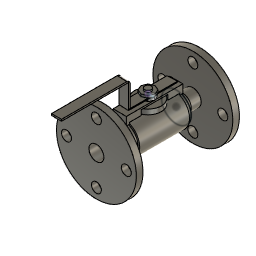
drawing 3 (pipe with handle) v5 (Autodesk Fusion 360 design; units mm, degrees)
Autodesk Fusion 360 part; units mm, degrees
sketch "Sketch1" plane through (0, 0, 0) normal (0, 0, 1) x (1, 0, 0)
  line L0 (0, -75) -> (0, 75)
  constraint vertical L0
pipe "Pipe1" add diameter 100 wall 5 path "Sketch1" along L0 makes body 1
sketch "Sketch2" plane through (0, 75, 0) normal (0, 1, 0) x (-1, 0, 0)
  circle A0 centre (0, 0) radius 45
  circle A1 centre (0, 0) radius 50
  circle A2 centre (0, 0) radius 45
  constraint coincident A0.centre A1.centre
extrude "Extrude1" add sketch "Sketch2" along normal blind 10 separate body contours A0 A2 makes body 2
sketch "Sketch3" plane through (0, 85, 0) normal (0, 1, 0) x (-1, 0, 0)
  circle A0 centre (0, 0) radius 45
  circle A1 centre (0, 0) radius 44
  dimension "d7" = 88
  constraint concentric A0 A1
  measures "d7" diameter of A1
hole "Hole1" at (0, 85, 0) direction (0, -1, 0) diameter 88 depth 40 tip angle 118 bodies 2
mirror "Mirror1" about plane through (0, 0, 0) normal (0, 1, 0) of "Extrude1" makes body 3
ref_plane "WorkPlane1" through (0, -85, 0) normal (0, 1, 0) x (0, 0, 1)
sketch "Sketch4" plane through (0, -85, 0) normal (0, -1, 0) x (1, 0, 0)
  circle A0 centre (0, 0) radius 45
  circle A1 centre (0, 0) radius 25
  dimension "d14" = 50
  constraint coincident A0.centre A1.centre
  measures "d14" diameter of A1
extrude "Extrude2" add sketch "Sketch4" along normal blind 50 contours A1 bodies 3
fillet "Fillet1" radius 20 1 edges at (-23.3082, -85, 9.0404) on bodies 3
ref_plane "WorkPlane2" through (0, -135, 0) normal (0, 1, 0) x (0, 0, 1)
hole "Hole2" at (0, -135, 0) direction (0, 1, 0) diameter 45 depth 60 tip angle 180 bodies 3
sketch "Sketch5" plane through (0, -135, 0) normal (0, 1, 0) x (1, 0, 0)
  circle A0 centre (0, 0) radius 120
  constraint coincident A0.centre origin
extrude "Extrude3" add sketch "Sketch5" against normal blind 20 bodies 3
hole "Hole3" at (0, -155, 0) direction (0, 1, 0) diameter 45 depth 20 tip angle 180 bodies 3
mirror "Mirror2" about plane through (0, 0, 0) normal (0, 1, 0) of bodies 3 makes body 4
sketch "Sketch6" plane through (0, 155, 0) normal (0, 1, 0) x (-1, 0, 0)
  circle A0 centre (0, 0) radius 22.5
  circle A1 centre (0, 0) radius 120
  circle A2 centre (0, 0) radius 90
  line L0 (0, 0) -> (90, 0)
  line L1 (0, 0) -> (0, 90)
  circle A3 centre (0, 90) radius 15
  circle A4 centre (90, 0) radius 15
  circle A5 centre (-90, 0) radius 15
  circle A6 centre (0, -90) radius 15
  dimension "d30" = 180
  dimension "d32" = 30
  dimension "d33" = 30
  dimension "d34" = 30
  dimension "d35" = 30
  constraint concentric A0 A2
  constraint coincident A0.centre A1.centre
  constraint coincident A2 L0.end
  constraint horizontal L0
  constraint coincident A2 L1.end
  constraint perpendicular L0 L1
  constraint coincident L1.end A3.centre
  constraint coincident L0.end A4.centre
  constraint coincident A2 A5.centre
  constraint coincident A2 A6.centre
  measures "d30" diameter of A2
  measures "d32" diameter of A3
  measures "d33" diameter of A4
  measures "d34" diameter of A5
  measures "d35" diameter of A6
extrude "Extrude4" cut sketch "Sketch6" against normal blind 20 contours A2 L0 A4 | A2 L0 A4 | A2 L1 A3 | A2 L1 A3 | A2 A4 | A2 A3 | A2 A6 | A2 A6 | A2 A5 | A2 A5 bodies 4
mirror "Mirror3" about plane through (0, 0, 0) normal (0, 1, 0) of "Extrude4"
mirror "Mirror4" about plane through (0, 0, 0) normal (0, 1, 0) of "Extrude4"
mirror "Mirror5" about plane through (0, 0, 0) normal (0, 1, 0) of "Extrude4"
sketch "Sketch7" plane through (0, -155, 0) normal (0, -1, 0) x (1, 0, 0)
  circle A0 centre (0, 0) radius 22.5
  circle A1 centre (0, 0) radius 120
  circle A2 centre (0, 0) radius 90
  circle A3 centre (0, 90) radius 15
  circle A4 centre (90, 0) radius 15
  circle A5 centre (0, -90) radius 15
  circle A6 centre (-90, 0) radius 15
  dimension "d44" = 180
  dimension "d45" = 30
  dimension "d46" = 30
  dimension "d47" = 30
  dimension "d48" = 30
  constraint concentric A0 A2
  constraint coincident A2 A3.centre
  constraint coincident A2 A4.centre
  constraint coincident A2 A5.centre
  constraint coincident A2 A6.centre
  measures "d44" diameter of A2
  measures "d45" diameter of A3
  measures "d46" diameter of A4
  measures "d47" diameter of A5
  measures "d48" diameter of A6
extrude "Extrude5" cut sketch "Sketch7" against normal blind 20 contours A2 A4 | A2 A4 | A2 A3 | A2 A3 | A2 A5 | A2 A5 | A2 A6 | A2 A6 bodies 3
ref_plane "WorkPlane3" through (0, 0, 50) normal (0, 0, 1) x (1, 0, 0)
sketch "Sketch8" plane through (0, 0, 50) normal (0, 0, 1) x (1, 0, 0)
  circle A0 centre (0, 0) radius 40
  constraint coincident A0.centre origin
extrude "Extrude6" add sketch "Sketch8" along normal blind 15 separate body makes body 5
ref_plane "WorkPlane1" through (0, -75, 0) normal (0, 1, 0) x (0, 0, 1) in component "handle"
sketch "Sketch1 (2)" plane through (0, -75, 0) normal (0, 1, 0) x (1, 0, 0) in component "handle"
ref_plane "WorkPlane4" through (0, 0, 50) normal (0, 0, 1) x (1, 0, 0)
ref_plane "WorkPlane5" through (0, 0, 60) normal (0, 0, 1) x (1, 0, 0)
sketch "Sketch9" plane through (0, 0, 60) normal (0, 0, 1) x (1, 0, 0)
  circle A0 through (40, 0, -10) (-20, 34.641, -10) (-20, -34.641, -10)
  line L0 (0, 40, 0) -> (0, 40, -10)
  circle A1 through (50, 75, -60) (-25, 75, -16.6987) (-25, 75, -103.3013)
  line L1 (0, 40, -10) -> (0, 75, -10)
  circle A2 through (45, 75, -60) (-22.5, 75, -21.0289) (-22.5, 75, -98.9711)
  line L2 (0, 75, -10) -> (0, 75, -15)
  circle A3 through (45, 85, -60) (-22.5, 85, -21.0289) (-22.5, 85, -98.9711)
  line L3 (0, 75, -15) -> (0, 85, -15)
  line L4 (0, 85, -15) -> (0, 85, 0)
  line L5 (0, 85) -> (0, 40)
  dimension "d57" = 15
  constraint vertical L5
extrude "Extrude7" add sketch "Sketch9" along normal mid plane 40 separate body contours L0 L1 L2 L3 L4 L5 in plane through (0, 0, 60) normal (1, 0, 0) makes body 6
mirror "Mirror6" about plane through (0, 0, 0) normal (0, 1, 0) of "Extrude7" makes body 7
move_face "OffsetFaces1" offset 10 2 faces at (6.6667, 70, 60) (6.6667, -70, 60) on bodies 6 7
sketch "Sketch10" plane through (0, 40, 0) normal (0, -1, 0) x (1, 0, 0)
  line L0 (-20, 50) -> (20, 50)
  line L1 (20, 50) -> (20, 70)
  line L2 (20, 70) -> (-20, 70)
  line L3 (-20, 70) -> (-20, 50)
  circle A0 through (40, 65, 40) (-20, 65, 74.641) (-20, 65, 5.359)
  line L4 (0, 65) -> (-20, 65)
  line L5 (-20, 70) -> (20, 70)
  line L6 (20, 65) -> (0, 65)
  constraint coincident L3 L4.end
  constraint perpendicular L3 L4
  constraint coincident L2.end L3.start
  constraint coincident L1.end L2.start
  constraint coincident L1 L6.start
extrude "Extrude8" add sketch "Sketch10" along normal blind 80 contours L1 L2 L3 L4 L5 L6 bodies 5 6 7
sketch "Sketch11" plane through (0, 0, 70) normal (0, 0, 1) x (-1, 0, 0)
  line L0 (20, -85) -> (20, 85)
  line L1 (20, 85) -> (-20, 85)
  line L2 (-20, 85) -> (-20, -85)
  line L3 (-20, -85) -> (20, -85)
  line L4 (14.1005, 14.0416) -> (0.0416, 19.8995)
  line L5 (0.0416, 19.8995) -> (-14.0416, 14.1005)
  line L6 (-14.0416, 14.1005) -> (-19.8995, 0.0416)
  line L7 (-19.8995, 0.0416) -> (-14.1005, -14.0416)
  line L8 (-14.1005, -14.0416) -> (-0.0416, -19.8995)
  line L9 (-0.0416, -19.8995) -> (14.0416, -14.1005)
  line L10 (14.0416, -14.1005) -> (19.8995, -0.0416)
  line L11 (19.8995, -0.0416) -> (14.1005, 14.0416)
extrude "Extrude9" add sketch "Sketch11" along normal blind 7 separate body contours L4 L5 L6 L7 L8 L9 L10 L11 makes body 8
sketch "Sketch12" plane through (0, 0, 77) normal (0, 0, 1) x (-1, 0, 0)
  line L0 (19.8995, -0.0416) -> (14.1005, 14.0416)
  line L1 (14.1005, 14.0416) -> (0.0416, 19.8995)
  line L2 (0.0416, 19.8995) -> (-14.0416, 14.1005)
  line L3 (-14.0416, 14.1005) -> (-19.8995, 0.0416)
  line L4 (-19.8995, 0.0416) -> (-14.1005, -14.0416)
  line L5 (-14.1005, -14.0416) -> (-0.0416, -19.8995)
  line L6 (-0.0416, -19.8995) -> (14.0416, -14.1005)
  line L7 (14.0416, -14.1005) -> (19.8995, -0.0416)
  line L8 (0, 0) -> (-15, 0)
  constraint coincident L8.start origin
ref_plane "WorkPlane9" through (0, 0, 77) normal (0, 0, 1) x (1, 0, 0)
sketch "Sketch13" plane through (0, 0, 77) normal (0, 0, 1) x (1, 0, 0)
  line L0 (0, 0) -> (-15, 0)
  line L1 (-15, 0) -> (-15, -72.1801)
  line L2 (15, 0) -> (15, -70)
  line L3 (15, -70) -> (15, -73.6216)
  line L4 (15, -73.6216) -> (-15, -72.1801)
  line L5 (-15, -72.1801) -> (15, -73.6216)
  line L6 (0, 0) -> (15, 0)
  point P0 (15, 0)
  constraint coincident L0.start L6.start
  constraint perpendicular L0 L1
  constraint coincident P0 L2.start
  constraint parallel L1 L2
  constraint parallel L2 L3
  constraint parallel L4 L5
  constraint perpendicular L2 L6
extrude "Extrude10" add sketch "Sketch13" along normal blind 3 bodies 8
mirror "Mirror7" about plane through (0, 0, 0) normal (0, 1, 0) of "Extrude10"
sketch "Sketch14" plane through (0, 0, 80) normal (0, 0, 1) x (-1, 0, 0)
  line L0 (15, -72.1801) -> (15, 72.1801)
  line L1 (15, 72.1801) -> (-15, 73.6216)
  line L2 (-15, 73.6216) -> (-15, -73.6216)
  line L3 (-15, -73.6216) -> (15, -72.1801)
  line L4 (21.3882, 0) -> (15.1237, 15.1237)
  line L5 (15.1237, 15.1237) -> (0, 21.3882)
  line L6 (0, 21.3882) -> (-15.1237, 15.1237)
  line L7 (-15.1237, 15.1237) -> (-21.3882, 0)
  line L8 (-21.3882, 0) -> (-15.1237, -15.1237)
  line L9 (-15.1237, -15.1237) -> (0, -21.3882)
  line L10 (0, -21.3882) -> (15.1237, -15.1237)
  line L11 (15.1237, -15.1237) -> (21.3882, 0)
extrude "Extrude11" add sketch "Sketch14" along normal blind 7 contours L0 L2 L5 L6 L9 L10 | L0 L4 L5 L10 L11 | L2 L6 L7 L8 L9 bodies 8
sketch "Sketch15" plane through (0, 0, 87) normal (0, 0, 1) x (-1, 0, 0)
  line L0 (15.1237, -15.1237) -> (21.3882, 0)
  line L1 (21.3882, 0) -> (15.1237, 15.1237)
  line L2 (15.1237, 15.1237) -> (0, 21.3882)
  line L3 (0, 21.3882) -> (-15.1237, 15.1237)
  line L4 (-15.1237, 15.1237) -> (-21.3882, 0)
  line L5 (-21.3882, 0) -> (-15.1237, -15.1237)
  line L6 (-15.1237, -15.1237) -> (0, -21.3882)
  line L7 (0, -21.3882) -> (15.1237, -15.1237)
  circle A0 centre (0, 0) radius 10
  constraint coincident A0.centre origin
extrude "Extrude12" add sketch "Sketch15" along normal blind 5 contours A0 bodies 8
sketch "Sketch16" plane through (0, 0, 80) normal (0, 0, 1) x (-1, 0, 0)
  line L0 (0, 21.3882) -> (15, 15.175)
  line L1 (15, 15.175) -> (15, 72.1801)
  line L2 (15, 72.1801) -> (-15, 73.6216)
  line L3 (-15, 73.6216) -> (-15, 15.175)
  line L4 (-15, 15.175) -> (0, 21.3882)
  line L5 (15, 72.1801, 0) -> (15, 72.1801, 70)
  line L6 (15, 72.1801, 70) -> (-10, 72.1801, 70)
  line L7 (-15, 73.6216, 0) -> (-15, 73.6216, 70)
  line L8 (15, 72.1801, 70) -> (-15, 73.6216, 70)
  line L9 (21.1406, 199.9755, 70) -> (-15, 199.9755, 70)
  line L10 (-15, 199.9755, 70) -> (-15, 73.6216, 70)
  line L11 (-15, 199.9755, 70) -> (-15, 400, 70)
  line L12 (-15, 400, 70) -> (-80, -250, 70)
  line L13 (-80, -250, 70) -> (-15, 400, 70)
  line L14 (-15, 400, 70) -> (15.015, 400, 70)
  line L15 (21.1406, 450, 70) -> (-15, 450, 70)
  line L16 (15, 72.1801, 70) -> (15, 199.9755, 70)
  line L17 (15, 199.9755, 70) -> (15.015, 400, 70)
  dimension "d81" = 70
  dimension "d82" = 70
  dimension "d83" = 30.015
  constraint coincident L1.end L2.start
  constraint coincident L2.end L3.start
  measures "d81" distance of L1.end L2.start
  measures "d82" distance of L2.end L3.start
extrude "Extrude13" add sketch "Sketch16" against normal blind 5 contours L2 L5 L7 L8 in plane through (-3.4948, -72.7329, 80) normal (-0.047995, -0.998848, 0) bodies 8
sketch "Sketch17" plane through (0, 0, 50) normal (0, 0, 1) x (1, 0, 0)
  line L0 (-15, -72.1801, 100) -> (-15, -275, 100)
  line L1 (15, -73.6216, 100) -> (15, -275, 100)
  line L2 (15, -275, 100) -> (-15, -275, 100)
  line L3 (15, -275, 100) -> (-15, -275, 100)
  line L4 (15, -275, 100) -> (-15, -275, 100)
  line L5 (15, -275, 100) -> (-15, -275, 100)
  line L6 (15, -275, 100) -> (-15, -275, 100)
  line L7 (15, -275, 100) -> (-15, -275, 100)
  line L8 (-15, -275, 100) -> (15, -275, 100)
  line L9 (-15, -72.1801, 100) -> (15, -73.6216, 100)
  point P0 (-15, -72.1801)
  point P1 (15, -73.6216)
extrude "Extrude14" add sketch "Sketch17" along normal blind 5 separate body contours L0 L1 L2 L3 L4 L5 L6 L7 L8 L9 in plane through (0, 0, 150) normal (0, 0, 1) makes body 9
sketch "Sketch18" plane through (0, 0, 150) normal (0, 0, 1) x (-1, 0, 0)
  line L0 (15, 72.1801) -> (-15, 73.6216)
  line L1 (-15, 73.6216) -> (-15.24, 68.6273)
  line L2 (-15.24, 68.6273) -> (14.76, 67.1859)
  line L3 (14.76, 67.1859) -> (15, 72.1801)
  line L4 (14.76, 67.1859) -> (-0.24, 67.9066)
  constraint coincident L2.end L3.start
  constraint midpoint L2 L4.end
extrude "Extrude15" add sketch "Sketch18" along normal blind 5 bodies 8 9
fillet "Fillet2" radius 10 1 edges at (0.24, -67.9066, 155) on bodies 8
component "handle" placed x (1, 0, 0) y (0, 1, 0) z (0, 0, 1) at (0, 0, 0)
